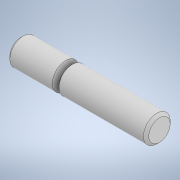
# Autodesk Inventor part: Втулка_Штрифта
Saved by Autodesk Inventor 2021 (Build 250183000, 183)
## iProperties
Created: 2023-04-15
Part Number: Втулка_Штрифта
Material: Типовые
Document SubType Name: Modeling
Designer: gdevc
Density: 1 g/cm^3
Appearance: По умолчанию
Author: gdevc
Autodesk Inventor part; units mm, degrees
ref_plane "YZ Plane" through (0, 0, 0) normal (1, 0, 0) x (0, 1, 0)
ref_plane "XZ Plane" through (0, 0, 0) normal (0, 1, 0) x (-1, 0, 0)
ref_plane "XY Plane" through (0, 0, 0) normal (0, 0, 1) x (1, 0, 0)
sketch "Эскиз1" plane through (0, 0, 0) normal (0, 0, 1) x (1, 0, 0)
  line L0 (0, 0) -> (52, 0)
  line L1 (0, 3) -> (50, 3)
  line L2 (0, 5) -> (0, 3)
  line L3 (52, 5) -> (52, 0)
  line L4 (50, 3) -> (50, 0)
  line L5 (16.892, 5) -> (18.142, 3.5103)
  line L6 (18.142, 3.5103) -> (19.392, 5)
  line L7 (0, 5) -> (16.892, 5)
  line L8 (19.392, 5) -> (52, 5)
  dimension "d0" = 6
  dimension "d1" = 52
  dimension "d4" = 2
  dimension "d5" = 16.892
  dimension "d11" = 2.5
  dimension "d12" = 50
  dimension "d13" = 50
  dimension "d14" = 10
  dimension "d15" = 10
  constraints: 18 end point, 4 horizontal, 2 point on line, 2 vertical, 1 perpendicular
  measures "d0" diameter of L1 L0
  measures "d1" distance of L0.start L0.end
  measures "d4" distance between parallel lines of L3 L4
  measures "d5" distance from line of L2 L5.start
  measures "d11" distance of L6.end L5.start
  measures "d12" angle of L7 L5
  measures "d13" angle of L8 L6
  measures "d14" diameter of L7 L0
  measures "d15" diameter of L8 L0
revolve "Вращение1" add sketch "Эскиз1" angle 360 about axis through (0, 0, 0) along (1, 0, 0)
chamfer "Фаска1" distance 1 angle 45 2 edges at (0, -5, 0) (52, -5, 0)
